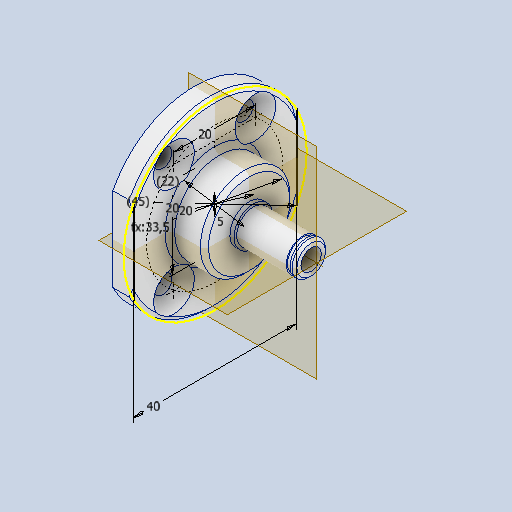
# Autodesk Inventor part: ParallelMecha_Supportlink_BottomShaft
Saved by Autodesk Inventor 2024 (Build 280153000, 153)
## iProperties
Created: 2022-08-03
Part Number: ParallelMecha_Supportlink_BottomShaft
Material: Aluminium 6061
Document SubType Name: Modeling
Designer: alexw
Density: 2.7 g/cm^3
Appearance: Aluminium - flach
Mass: 28.0828 g
Surface Area: 51.0383 cm^2
Volume: 10.401 cm^3
SupportFixation_HoleDia: 20,000 mm
Anlaufscheibe_JTM_1018_Thickness: 1,000 mm
Author: alexw
Autodesk Inventor part; units mm, degrees
ref_plane "YZ Plane" through (0, 0, 0) normal (1, 0, 0) x (0, 1, 0)
sketch "Skizze1" plane through (0, 0, 0) normal (0, 0, 1) x (1, 0, 0)
  line L0 (0, 0) -> (0, 22.5)
  line L1 (0, 22.5) -> (5, 22.5)
  line L2 (13.5, 11) -> (13.5, 4.75)
  line L3 (13.5, 4.75) -> (14.5, 4.75)
  line L4 (14.5, 4.75) -> (14.5, 4)
  line L5 (14.5, 4) -> (26.7, 4)
  line L6 (26.7, 4) -> (26.7, 3.8)
  line L7 (26.7, 3.8) -> (27.6, 3.8)
  line L8 (27.6, 3.8) -> (27.6, 4)
  line L9 (27.6, 4) -> (28.2, 4)
  line L10 (28.7, 3.5) -> (28.7, 0)
  line L11 (28.7, 0) -> (0, 0)
  line L12 (28.2, 4) -> (28.7, 3.5)
  line L13 (26.7, 4) -> (26.7, 0) construction
  line L14 (14.5, 4) -> (14.5, 0) construction
  line L15 (20.6, 4) -> (20.6, 0) construction
  line L16 (15.6, 4) -> (15.6, 0) construction
  line L17 (25.6, 4) -> (25.6, 0) construction
  line L18 (0, 8) -> (13.5, 8) construction
  line L19 (0, 12) -> (13.5, 12) construction
  line L20 (19.5, 4) -> (19.5, 0) construction
  line L21 (13.5, 10) -> (0, 10) construction
  line L22 (5, 22.5) -> (5, 11)
  line L23 (5, 11) -> (13.5, 11)
  point P0 (28.7, 4)
  dimension "d0" = 8
  dimension "d1" = 7.6
  dimension "d2" = 0.9
  dimension "d3" = 0.5
  dimension "d4" = 0.5
  dimension "d5" = 0.6
  dimension "d9" = 1.1
  dimension "d10" = 1.1
  dimension "d11" = 9.5
  dimension "d13" = 1
  dimension "SupportJoint_Proximal_Thickness" = 13.5
  dimension "d17" = 4
  dimension "d33" = 5
  dimension "d34" = 5
  dimension "d35" = 10
  dimension "d36" = 2
  dimension "d38" = 20
  dimension "d42" = 45
  dimension "d45" = 22
  dimension "d46" = 5
  constraints: 46 end point, 17 perpendicular, 14 point on line, 4 vertical, 1 collinear, 1 parallel, 10 other
  measures "d1" diameter of L7 L11
  measures "d2" distance between parallel lines of L8 L6
  measures "d3" distance of L9.end point (28.7, 4)
  measures "d4" distance of L10.start point (28.7, 4)
  measures "d5" distance from line of L8 L9.end
  measures "d9" distance between parallel lines of L14 L16
  measures "d10" distance between parallel lines of L17 L13
  measures "d11" diameter of L3 L11
  measures "d13" distance between parallel lines of L2 L14
  measures "SupportJoint_Proximal_Thickness" distance between parallel lines of L0 L2
  measures "d17" distance between parallel lines of L19 L18
  measures "d33" distance between parallel lines of L15 L17
  measures "d34" distance between parallel lines of L14 L20
  measures "d35" distance between parallel lines of L17 L16
  measures "d36" distance between parallel lines of L19 L21
  measures "d38" diameter of L21 L11
  measures "d42" diameter of L1 L11
  measures "d45" diameter of L23 L11
  measures "d46" distance between parallel lines of L0 L22
revolve "Umdrehung1" add sketch "Skizze1" angle 360 about axis through (28.7, 0, 0) along (-1, 0, 0)
sketch "Skizze2" plane through (5, 0, 0) normal (1, 0, 0) x (0, 0, -1)
  circle A0 centre (0, 0) radius 11 construction
  circle A1 centre (0, 0) radius 4.75 projected
  circle A2 centre (0, 0) radius 11 construction
  line L0 (-4.5826, 10) -> (4.5826, 10)
  line L1 (-4.5826, -10) -> (4.5826, -10)
  circle A3 centre (0, 0) radius 10 construction
  line L2 (-10, 0) -> (10, 0) construction
  line L3 (-10, 13.4374) -> (10, 13.4374) construction
  line L4 (0, 0) -> (0, 13.4374) construction
  circle A4 centre (0, 0) radius 3.5 construction
  circle A5 centre (0, 0) radius 16.75 construction
  circle A6 centre (0, 0) radius 22.5 projected
  line L5 (-20, -10.3078) -> (-20, 10.3078)
  line L6 (20, -10.3078) -> (20, 10.3078)
  circle A7 centre (0, 0) radius 2.5
  point P0 (4.5826, -10)
  point P1 (-4.5826, -10)
  point P2 (-4.5826, 10)
  point P3 (4.5826, 10)
  point P4 (-10, -13.4374)
  point P5 (10, -13.4374)
  dimension "d49" = 33.5
  dimension "d21" = 20
  dimension "d24" = 22
  dimension "SupportFixation_HoleDia" = 20
  dimension "d47" = 20
  dimension "d48" = 45
  dimension "d50" = 40
  dimension "d66" = 5
  constraints: 14 end point, 10 point on circle, 4 horizontal, 3 coincident, 3 parallel, 2 centre point, 2 midpoint, 2 symmetric about line, 2 vertical, 3 other
  measures "d21" distance between parallel lines of L0 L1
  measures "d24" diameter of A0
  measures "SupportFixation_HoleDia" diameter of A3
  measures "d47" distance of L3.start L3.end
  measures "d48" diameter of A6
  measures "d50" distance between parallel lines of L5 L6
  measures "d66" diameter of A7
extrude "Extrusion3" cut sketch "Skizze2" against normal through all contours A6 L6 | L5 A6
hole "Bohrung2" at (5, 13.4374, 10) at (5, 13.4374, -10) at (5, -13.4374, 10) at (5, -13.4374, -10) direction (-1, 0, 0) diameter 4.5 end through all countersink diameter 10 countersink angle 90 clearance for "Innensechskant-Senkkopfschraube DIN EN ISO 10642" size "M4" standard "DIN"
chamfer "Fase1" distance 1 angle 45 3 edges at (13.5, -11, 0) (5, -22.5, 0) (5, 22.5, 0)
fillet "Rundung1" radius 1.2 1 edges at (5, -11, 0)
thicken "Verdickung1" operation add thickness 0.1 both sides no extend neighbours yes toward (0, 0.9870503, 0.1604113) faces at (22.6333, 3.9482, 0.6416) (28, 3.987, 0.3219)
extrude "Extrusion4" cut sketch "Skizze2" along normal through all both and the other way through all contours A7
equation "\"d49\" = 0.5 * d48 + 0.5 * d24"
equation "\"d4\" = d3"
equation "\"d10\" = d9"
equation "\"d13\" = Anlaufscheibe_JTM_1018_Thickness"
equation "\"d34\" = d33"
equation "\"d36\" = 0.5 * d17"
equation "\"Anlaufscheibe_JTM_1018_Thickness\" = 1"
